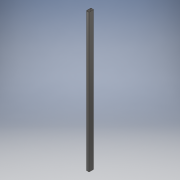
# Autodesk Inventor part: 1.5 X 2.5 X .125 WALL SQ TUBE-03
Saved by Autodesk Inventor 2018.2 (Build 222227000, 227)
## iProperties
Created: 2017-12-10
Part Number: 1.5 X 2.5 X .125 WALL SQ TUBE-03
Material: Steel
Document SubType Name: Modeling
Designer: torba
Density: 7.85 g/cm^3
Appearance: Steel - Polished
Author: torba
Autodesk Inventor part; units mm, degrees
ref_plane "YZ Plane" through (0, 0, 0) normal (1, 0, 0) x (0, 1, 0)
ref_plane "XZ Plane" through (0, 0, 0) normal (0, 1, 0) x (-1, 0, 0)
ref_plane "XY Plane" through (0, 0, 0) normal (0, 0, 1) x (1, 0, 0)
sketch "Sketch1" plane through (0, 0, 0) normal (0, 1, 0) x (-1, 0, 0)
  line L0 (0, 0) -> (38.1, 0)
  line L1 (38.1, 0) -> (38.1, -63.5)
  line L2 (38.1, -63.5) -> (0, -63.5)
  line L3 (0, -63.5) -> (0, 0)
  line L4 (34.925, -3.175) -> (3.175, -3.175)
  line L5 (3.175, -3.175) -> (3.175, -60.325)
  line L6 (3.175, -60.325) -> (34.925, -60.325)
  line L7 (34.925, -60.325) -> (34.925, -3.175)
  dimension "d0" = 38.1
  dimension "d1" = 63.5
  dimension "d2" = 3.175
  dimension "d3" = 3.175
  dimension "d4" = 3.175
  dimension "d5" = 3.175
  constraints: 16 end point, 4 parallel, 2 horizontal, 2 perpendicular
  measures "d0" distance of L1.end L2.end
  measures "d1" distance of L0.end L1.end
  measures "d2" distance between parallel lines of L3 L5
  measures "d3" distance between parallel lines of L0 L4
  measures "d4" distance between parallel lines of L1 L7
  measures "d5" distance between parallel lines of L2 L6
extrude "Extrusion1" add sketch "Sketch1" along normal blind 1828.8
fillet "Fillet1" radius 3.175 8 edges at (-34.925, 914.4, -3.175) (-38.1, 914.4, 0) (-38.1, 914.4, -63.5) (-34.925, 914.4, -60.325) (0, 914.4, -63.5) (-3.175, 914.4, -60.325) (0, 914.4, 0) (-3.175, 914.4, -3.175)
equation "\"d3\" = d2"
equation "\"d4\" = d2"
equation "\"d5\" = d2"
body "Solid1"
